Autodesk Inventor part; units mm, degrees
(part 2 of 2)
extrude "REF_PADS_DIAGONAL" add sketch "REF_PADS_DRAW" along normal blind 0.1 separate body
sketch "ref_pad_back_draw" plane through (0, 0, 0) normal (0, 0, -1) x (-1, 0, 0)
  circle A0 centre (9.4953, -6.3108) radius 1.3847
  arc A1 (9.0004, -6.0033) -> (9.2004, -5.8033) centre (9.0004, -5.8033) ccw projected
  circle A2 centre (9.4953, -6.3108) radius 0.7089
  point P0 (0, 0)
  constraints: 1 centre point, 1 coincident, 3 other
extrude "REF_PAD_BACK" add sketch "ref_pad_back_draw" along normal blind 0.1 separate body
equation "\"d8\" = d7"
